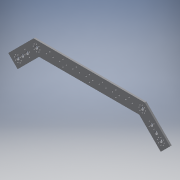
# Autodesk Inventor part: KrakenCsideplate1
Saved by Autodesk Inventor 2016 (Build 200138000, 138)
## iProperties
Created: 2015-09-13
Part Number: KrakenCsideplate1
Material: Generic
Document SubType Name: Modeling
Designer: Tim
Density: 1 g/cm^3
Appearance: Default
Author: Tim
Autodesk Inventor part; units mm, degrees
ref_plane "YZ Plane" through (0, 0, 0) normal (1, 0, 0) x (0, 1, 0)
ref_plane "XZ Plane" through (0, 0, 0) normal (0, 1, 0) x (-1, 0, 0)
ref_plane "XY Plane" through (0, 0, 0) normal (0, 0, 1) x (1, 0, 0)
sketch "Sketch1" plane through (0, 0, 0) normal (0, 0, 1) x (1, 0, 0)
  line L0 (-41.0226, 338.1145) -> (-60.1145, 319.0226)
  line L1 (-10, 66.5) -> (-10, 221.5)
  circle A0 centre (-22.2843, 288.9706) radius 1.85
  circle A1 centre (-10.9706, 288.9706) radius 1.85
  circle A2 centre (-10.9706, 300.2843) radius 1.85
  circle A3 centre (-16.6274, 294.6274) radius 4
  circle A4 centre (-22.2843, 300.2843) radius 1.85
  circle A5 centre (-27.9411, 305.9411) radius 4
  circle A6 centre (-31.2548, 317.2548) radius 1.85
  circle A7 centre (-33.598, 322.9117) radius 1.85
  circle A8 centre (-39.2548, 325.2548) radius 1.85
  circle A9 centre (-39.2548, 317.2548) radius 4
  circle A10 centre (-33.598, 311.598) radius 1.85
  circle A11 centre (-39.2548, 309.2548) radius 1.85
  circle A12 centre (-44.9117, 311.598) radius 1.85
  circle A13 centre (-47.2548, 317.2548) radius 1.85
  circle A14 centre (-44.9117, 322.9117) radius 1.85
  circle A15 centre (6, 272) radius 4
  circle A16 centre (11.6569, 277.6569) radius 1.85
  circle A17 centre (6, 280) radius 1.85
  circle A18 centre (14, 272) radius 1.85
  circle A19 centre (11.6569, 266.3431) radius 1.85
  circle A20 centre (6, 264) radius 1.85
  circle A21 centre (0.3431, 266.3431) radius 1.85
  circle A22 centre (-2, 272) radius 1.85
  circle A23 centre (0.3431, 277.6569) radius 1.85
  circle A24 centre (6, 248) radius 1.85
  circle A25 centre (6, 232) radius 1.85
  circle A26 centre (6, 216) radius 1.85
  circle A27 centre (6, 200) radius 1.85
  circle A28 centre (6, 184) radius 1.85
  circle A29 centre (6, 168) radius 1.85
  circle A30 centre (6, 8) radius 1.85
  circle A31 centre (6, 24) radius 1.85
  circle A32 centre (6, 40) radius 1.85
  circle A33 centre (6, 56) radius 1.85
  circle A34 centre (6, 72) radius 1.85
  circle A35 centre (6, 88) radius 1.85
  circle A36 centre (6, 104) radius 1.85
  circle A37 centre (6, 120) radius 1.85
  circle A38 centre (6, 136) radius 1.85
  circle A39 centre (6, 152) radius 1.85
  circle A40 centre (14, 16) radius 1.85
  circle A41 centre (11.6569, 21.6569) radius 1.85
  circle A42 centre (11.6569, 10.3431) radius 1.85
  circle A43 centre (6, 16) radius 4
  circle A44 centre (0.3431, 10.3431) radius 1.85
  circle A45 centre (-2, 16) radius 1.85
  circle A46 centre (0.3431, 21.6569) radius 1.85
  line L2 (-41.0226, -50.1145) -> (-60.1145, -31.0226)
  circle A47 centre (-31.2548, -29.2548) radius 1.85
  circle A48 centre (-33.598, -34.9117) radius 1.85
  circle A49 centre (-39.2548, -37.2548) radius 1.85
  circle A50 centre (-33.598, -23.598) radius 1.85
  circle A51 centre (-39.2548, -21.2548) radius 1.85
  circle A52 centre (-44.9117, -23.598) radius 1.85
  circle A53 centre (-44.9117, -34.9117) radius 1.85
  circle A54 centre (-47.2548, -29.2548) radius 1.85
  circle A55 centre (-39.2548, -29.2548) radius 4
  circle A56 centre (-22.2843, -12.2843) radius 1.85
  circle A57 centre (-27.9411, -17.9411) radius 4
  circle A58 centre (-10.9706, -12.2843) radius 1.85
  circle A59 centre (-10.9706, -0.9706) radius 1.85
  circle A60 centre (-16.6274, -6.6274) radius 4
  circle A61 centre (-22.2843, -0.9706) radius 1.85
  line L3 (-10, 221.5) -> (-10, 265.3726)
  line L4 (-10, 66.5) -> (-10, 22.6274)
  line L5 (-61.8823, -29.2548) -> (-60.1145, -31.0226)
  line L6 (-41.0226, -50.1145) -> (-39.2548, -51.8823)
  line L7 (-60.1145, 319.0226) -> (-61.8823, 317.2548)
  line L8 (-39.2548, 339.8823) -> (-41.0226, 338.1145)
  line L9 (-10, 22.6274) -> (-61.8823, -29.2548)
  line L10 (-10, 265.3726) -> (-61.8823, 317.2548)
  circle A62 centre (14, 112) radius 1.85 projected
  circle A63 centre (14, 144) radius 1.85 projected
  circle A64 centre (14, 176) radius 1.85 projected
  circle A65 centre (14, 208) radius 1.85 projected
  circle A66 centre (14, 240) radius 1.85 projected
  circle A67 centre (14, 80) radius 1.85 projected
  circle A68 centre (14, 48) radius 1.85 projected
  circle A69 centre (-2, 208) radius 1.85 projected
  circle A70 centre (-2, 144) radius 1.85 projected
  circle A71 centre (-2, 80) radius 1.85 projected
  line L11 (-39.2548, 339.8823) -> (22, 278.6274)
  line L12 (-39.2548, -51.8823) -> (22, 9.3726)
  line L13 (22, 278.6274) -> (22, 9.3726)
  point P0 (0, 0)
  constraints: 62 centre point, 28 end point, 3 perpendicular, 2 point on line, 1 collinear, 1 parallel, 1 vertical
extrude "Extrusion2" add sketch "Sketch1" along normal blind 4
body "Solid2"
